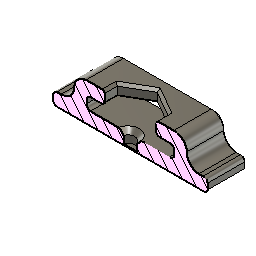
BeltClip (Autodesk Fusion 360 design; units mm, degrees)
Autodesk Fusion 360 part; units mm, degrees
sketch "Sketch1" plane through (0, 0, 0) normal (0, 0, 1) x (1, 0, 0)
  line L0 (0, 3) -> (10.5, 3)
  line L1 (10.5, 3) -> (10.5, 0)
  line L2 (10.5, 0) -> (0, 0)
  line L3 (0, 6) -> (13.5, 6)
  line L4 (13.5, 6) -> (13.5, 0)
  line L5 (13.5, 0) -> (18.5, 0)
  line L6 (18.5, 0) -> (18.5, -3)
  line L7 (18.5, -3) -> (0, -3)
  line L8 (0, 6) -> (0, 3)
  line L9 (0, -3) -> (0, 0)
  dimension "d1" = 10.5
  dimension "d2" = 3
  dimension "d3" = 3
  dimension "d4" = 6
  dimension "d5" = 3
  dimension "d6" = 5
  constraint horizontal L0
  constraint perpendicular L0 L1
  constraint coincident L2.end L9.end
  constraint perpendicular L1 L2
  constraint parallel L0 L3
  constraint perpendicular L0 L4
  constraint perpendicular L4 L5
  constraint perpendicular L0 L6
  constraint perpendicular L6 L7
  constraint collinear L2 L5
  constraint perpendicular L0 L8
  constraint perpendicular L2 L9
  constraint collinear L8 L9
  measures "d1" distance of L1.end L2.end
  measures "d2" distance of L5.end L6.end
  measures "d3" distance of L0.end L1.end
  measures "d4" distance of L3.end L4.end
  measures "d5" distance of L1 L4
  measures "d6" distance of L4.end L5.end
extrude "Extrude1" add sketch "Sketch1" along normal blind 20
fillet "Fillet1" radius 1 2 edges at (10.5, 3, 10) (10.5, 0, 10)
fillet "Fillet1" radius 3 2 edges at (13.5, 6, 10) (13.5, 0, 10)
fillet "Fillet1" radius 1 1 edges at (18.5, 0, 10)
mirror "Mirror1" about plane through (0, -3, 0) normal (-1, 0, 0) of bodies 1 merged
chamfer "Chamfer1" distance 0.6 angle 45 2 faces at (-3.1667, -2, 20) (-3.1667, -2, 0)
chamfer "Chamfer1" distance 0.6 angle 45 2 edges at (18.5, -3, 10) (-18.5, -3, 10)
sketch "Sketch2" plane through (0, 6, 0) normal (0, 1, 0) x (-1, 0, 0)
  line L0 (10.5, 19.4) -> (-10.5, 19.4)
  line L1 (-10.5, 19.4) -> (-10.5, 0.6)
  line L2 (-10.5, 0.6) -> (10.5, 0.6)
  line L3 (10.5, 0.6) -> (10.5, 19.4)
  line L4 (-10.5, 0.6) -> (10.5, 19.4) construction
  line L5 (-6.0622, 13.5) -> (-6.0622, 6.5)
  line L6 (-6.0622, 6.5) -> (0, 3)
  line L7 (0, 3) -> (6.0622, 6.5)
  line L8 (6.0622, 6.5) -> (6.0622, 13.5)
  line L9 (6.0622, 13.5) -> (0, 17)
  line L10 (0, 17) -> (-6.0622, 13.5)
  point P0 (0, 10)
  point P1 (0, 10)
  dimension "d19" = 7
  constraint coincident L1.end L2.start
  constraint coincident L0.start L3.end
  constraint midpoint L4 P1
  constraint coincident P1 P0
  constraint vertical origin L6.end
  measures "d19" distance of L7.end P1
extrude "Extrude2" cut sketch "Sketch2" against normal up to surface (3 mm away) contours L5 L6 L7 L8 L9 L10
chamfer "Chamfer2" distance 0.6 angle 45 12 edges at (-3.0311, 6, 4.75) (-6.0622, 6, 10) (-3.0311, 6, 15.25) (3.0311, 6, 15.25) (6.0622, 6, 10) (3.0311, 6, 4.75) (-3.0311, 3, 4.75) (3.0311, 3, 4.75) (6.0622, 3, 10) (3.0311, 3, 15.25) (-3.0311, 3, 15.25) (-6.0622, 3, 10)
hole "Hole1" at (0, 0, 10) direction (0, -1, 0) diameter 3.3 depth 2.8 tip angle 180 countersink diameter 5.5 countersink angle 90
equation "d1 = ( 21 / 2 ) * 1 mm"
equation "d3 = d2"
equation "d4 = 2 * d2"
equation "d5 = d2"
named bodies: "BeltClip"
